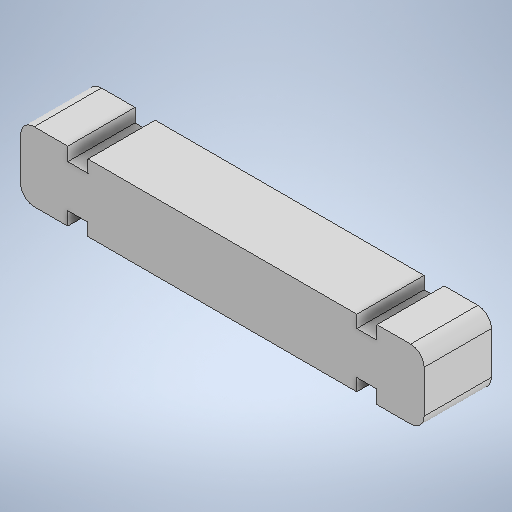
# Autodesk Inventor part: zebro_ac30_8
Saved by Autodesk Inventor 2025 (Build 290162000, 162)
## iProperties
Created: 2025-01-11
Part Number: zebro_ac30_8
Material: Všeobecné
Document SubType Name: Modeling
Designer: lukas
Density: 1 g/cm^3
Appearance: Výchozí
Author: lukas
## iProperties of the stored document zebro_ac30_8_3D tisk.ipt
Created: 2025-01-11
Part Number: zebro_ac30_8_3D tisk
Material: Všeobecné
Document SubType Name: Modeling
Designer: lukas
Density: 1 g/cm^3
Appearance: Výchozí
Author: lukas
Autodesk Inventor part; units mm, degrees
ref_plane "YZ Plane" through (0, 0, 0) normal (1, 0, 0) x (0, 1, 0)
ref_plane "XZ Plane" through (0, 0, 0) normal (0, 1, 0) x (-1, 0, 0)
ref_plane "XY Plane" through (0, 0, 0) normal (0, 0, 1) x (1, 0, 0)
sketch "Náčrt1" plane through (0, 0, 0) normal (0, 0, 1) x (1, 0, 0)
  line L0 (0, 7) -> (0, -7) projected
  line L1 (-28, 0) -> (28, 0) projected
  line L2 (-20, 5) -> (20, 5)
  line L3 (20, 5) -> (20, -5)
  line L4 (20, -5) -> (-20, -5)
  line L5 (-20, -5) -> (-20, 5)
  point P0 (0, 0)
  dimension "d0" = 10
  dimension "d1" = 40
  constraints: 8 end point, 2 parallel, 1 horizontal, 1 perpendicular, 2 other
  measures "d0" distance of L2.end L3.end
  measures "d1" distance of L2.start L2.end
extrude "Vysunutí1" add sketch "Náčrt1" along normal blind 10
sketch "Náčrt3" plane through (0, 0, 0) normal (0, 0, 1) x (1, 0, 0)
  line L0 (-5.5828, 0) -> (15.9971, 0) projected
  line L1 (0, -7.7899) -> (0, 7.7899) projected
  line L2 (-20, -5) -> (20, -5) projected
  line L3 (-20, 5) -> (-20, -5) projected
  line L4 (20, 5) -> (-20, 5) projected
  line L5 (20, -5) -> (20, 5) projected
  line L6 (20, 3.15) -> (23, 3.15)
  line L7 (23, 3.15) -> (23, 5.15)
  line L8 (23, 5.15) -> (28, 5.15)
  line L9 (30, 3.15) -> (30, 0)
  line L10 (-5.5828, 0) -> (15.9971, 0) projected
  line L11 (20, 3.15) -> (20, 0)
  line L12 (20, -5) -> (20, 5) projected
  line L13 (20, -3.15) -> (23, -3.15)
  line L14 (23, -3.15) -> (23, -5.15)
  line L15 (23, -5.15) -> (28, -5.15)
  line L16 (30, -3.15) -> (30, 0)
  line L17 (20, -3.15) -> (20, 0)
  arc A0 (30, 3.15) -> (28, 5.15) centre (28, 3.15) ccw
  arc A1 (28, -5.15) -> (30, -3.15) centre (28, -3.15) ccw
  line L18 (-20, 3.15) -> (-23, 3.15)
  line L19 (-23, 3.15) -> (-23, 5.15)
  line L20 (-23, 5.15) -> (-28, 5.15)
  line L21 (-30, 3.15) -> (-30, 0)
  line L22 (-20, 3.15) -> (-20, 0)
  line L23 (-20, -3.15) -> (-23, -3.15)
  line L24 (-23, -3.15) -> (-23, -5.15)
  line L25 (-23, -5.15) -> (-28, -5.15)
  line L26 (-30, -3.15) -> (-30, 0)
  line L27 (-20, -3.15) -> (-20, 0)
  arc A2 (-28, 5.15) -> (-30, 3.15) centre (-28, 3.15) ccw
  arc A3 (-30, -3.15) -> (-28, -5.15) centre (-28, -3.15) ccw
  point P0 (0, 0)
  point P1 (30, 5.15)
  point P2 (30, -5.15)
  dimension "d6" = 3
  dimension "d7" = 2
  dimension "d8" = 7
  dimension "d9" = 5.15
  dimension "d10" = 2
  dimension "d11" = 2
  constraints: 40 end point, 18 symmetric about line, 8 point on circle, 6 point on line, 4 centre point, 4 tangent, 3 perpendicular, 1 collinear, 1 horizontal, 1 midpoint, 2 other
  measures "d6" distance of L6.start L6.end
  measures "d7" distance of L6.end L7.end
  measures "d8" distance of L7.end point (30, 5.15)
  measures "d9" distance of point (30, 5.15) L9.end
  measures "d10" radius of A0
  measures "d11" radius of A1
extrude "Vysunutí2" add sketch "Náčrt3" along normal blind 10 contours L23 L24 L25 A3 L26 L21 A2 L20 L19 L18 L3 | L5 L6 L7 L8 A0 L9 L16 A1 L15 L14 L13
